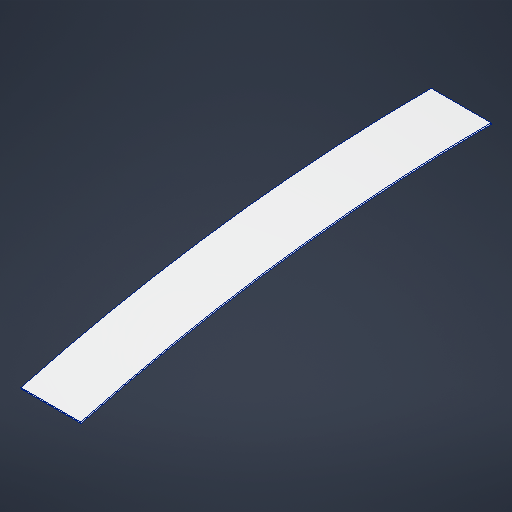
# Autodesk Inventor part: Doubler Plate
Saved by Autodesk Inventor 2026.2 (Build 302298000, 298)
## iProperties
Created: 2026-02-03
Part Number: Doubler Plate
Material: Aluminum 6061
Document SubType Name: Modeling
Designer: Lex Machina
Density: 2.7 g/cm^3
Appearance: Aluminum - Flat
Author: Lex Machina
Autodesk Inventor part; units mm, degrees
ref_plane "YZ Plane" through (0, 0, 0) normal (1, 0, 0) x (0, 1, 0)
ref_plane "XZ Plane" through (0, 0, 0) normal (0, 1, 0) x (-1, 0, 0)
ref_plane "XY Plane" through (0, 0, 0) normal (0, 0, 1) x (1, 0, 0)
sketch "Sketch1" plane through (0, 0, 0) normal (0, 0, 1) x (1, 0, 0)
  line L0 (0, 0) -> (80, 0)
  line L1 (80, 0) -> (80, 2)
  line L2 (80, 2) -> (0, 2)
  line L3 (0, 2) -> (0, 0)
  dimension "d0" = 80
  dimension "d1" = 2
  constraints: 8 end point, 2 parallel, 1 horizontal, 1 perpendicular
  measures "d0" distance of L2.end L1.end
  measures "d1" distance of L1.end L0.end
sketch "Sketch2" plane through (0, 0, 0) normal (1, 0, 0) x (0, 1, 0)
  line L0 (0, 0) -> (-2118, 0) construction
  arc A0 (0, 0) -> (-72.1691, 548.1787) centre (-2118, 0) ccw
  line L1 (-2118, 0) -> (-72.1691, 548.1787) construction
  line L2 (-2118, 0) -> (0, 0) construction
  dimension "d2" = 2118
  dimension "d3" = 15
  constraints: 6 end point, 2 point on circle, 1 centre point, 1 coincident, 1 horizontal
  measures "d2" distance of L0.start L0.end
  measures "d3" angle of L2 L1
sweep "Sweep1" add profiles "Sketch1" path "Sketch2"
body "Solid1"
